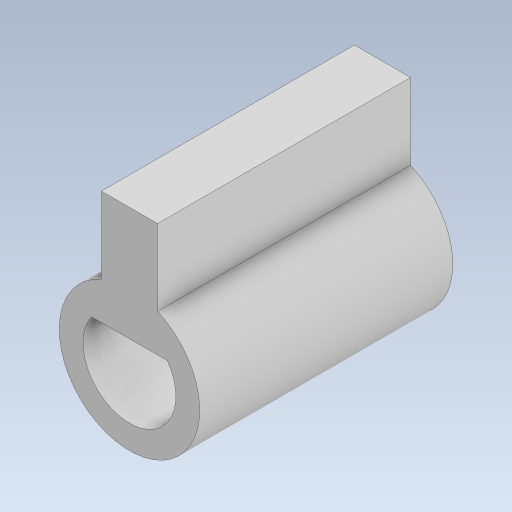
# Autodesk Inventor part: As Lifter
Saved by Autodesk Inventor 2023.5 (Build 275446000, 446)
## iProperties
Created: 2025-09-02
Part Number: As Lifter
Material: Generic
Document SubType Name: Modeling
Designer: Guntur
Density: 1 g/cm^3
Appearance: Default
Author: Guntur
## iProperties of the stored document As Lifter_3DPrint.ipt
Created: 2025-09-02
Part Number: As Lifter_3DPrint
Material: Generic
Document SubType Name: Modeling
Designer: Guntur
Density: 1 g/cm^3
Appearance: Default
Author: Guntur
Autodesk Inventor part; units mm, degrees
ref_plane "YZ Plane" through (0, 0, 0) normal (1, 0, 0) x (0, 1, 0)
ref_plane "XZ Plane" through (0, 0, 0) normal (0, 1, 0) x (-1, 0, 0)
ref_plane "XY Plane" through (0, 0, 0) normal (0, 0, 1) x (1, 0, 0)
sketch "Sketch1" plane through (0, 0, 0) normal (0, 0, 1) x (1, 0, 0)
  arc A0 (1, -9.9499) -> (-1, -9.9499) centre (0, 0) ccw
  line L0 (1, -11) -> (1, -9.9499)
  line L1 (-1, -11) -> (-1, -9.9499)
  arc A1 (-1.3491, 0.95) -> (1.3491, 0.95) centre (0, 0) ccw
  line L2 (0, 0.95) -> (1.3491, 0.95)
  line L3 (0, 0.95) -> (-1.3491, 0.95)
  line L4 (-1, -11) -> (-1, -12)
  line L5 (-1, -12) -> (1, -12)
  line L6 (1, -12) -> (1, -11)
  circle A2 centre (0, 0) radius 2.5
  line L7 (-1, 5) -> (1, 5)
  line L8 (1, 5) -> (1, 0)
  line L9 (1, 0) -> (-1, 0)
  line L10 (-1, 0) -> (-1, 5)
  line L11 (-1, 5) -> (1, 0) construction
  line L12 (1, 5) -> (-1, 0) construction
  point P0 (0, 2.5)
  point P1 (-1, 2.2913)
  point P2 (1, 2.2913)
  dimension "d29" = 5
  dimension "d16" = 3.3
  dimension "d18" = 1
  dimension "d30" = 2
  dimension "d31" = 5
  constraints: 26 end point, 4 point on circle, 3 perpendicular, 2 centre point, 2 coincident, 2 horizontal, 2 midpoint, 2 parallel, 1 point on line, 1 vertical, 3 other
  measures "d16" diameter of A1
  measures "d18" distance of L1.start L4.end
  measures "d30" distance of L8.end L9.end
  measures "d31" distance of L7.end L8.end
extrude "Extrusion1" add sketch "Sketch1" along normal blind 9 contours A1 L2 L8 A2 L10 L3 | L10 A2 L8 L2 L3 | L10 L7 L8 A2
body "Solid1"
